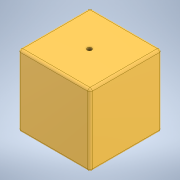
# Autodesk Inventor part: 1x2 Block v2
Saved by Autodesk Inventor 2020.1 (Build 241239000, 239)
## iProperties
Created: 2019-09-13
Part Number: 1x2 Block v2
Material: Generic
Document SubType Name: Modeling
Designer: alpha
Density: 1 g/cm^3
Appearance: Default
Author: alpha
Revision Number: ANY
Autodesk Inventor part; units mm, degrees
ref_plane "YZ Plane" through (0, 0, 0) normal (1, 0, 0) x (0, 1, 0)
ref_plane "XZ Plane" through (0, 0, 0) normal (0, 1, 0) x (-1, 0, 0)
ref_plane "XY Plane" through (0, 0, 0) normal (0, 0, 1) x (1, 0, 0)
ref_plane "Work Plane3" through (101.6, 2.54, 38.1) normal (1, 0, 0) x (0, 0, -1)
sketch "Sketch1" plane through (101.6, 2.54, 38.1) normal (1, 0, 0) x (0, 0, -1)
  line L0 (88.9, -2.54) -> (-12.7, -2.54)
  line L1 (-12.7, -2.54) -> (-12.7, 99.06)
  line L2 (-12.7, 99.06) -> (88.9, 99.06)
  line L3 (88.9, 99.06) -> (88.9, -2.54)
  point P0 (38.1, -2.54)
  constraints: 8 end point, 2 parallel, 1 horizontal, 1 perpendicular
extrude "Extrusion1" add sketch "Sketch1" along normal blind 101.6
sketch "Sketch2" plane through (101.6, 0, -50.8) normal (0, -1, 0) x (1, 0, 0)
  circle A0 centre (50.8, 50.8) radius 34.29
  point P0 (-101.6, 50.8)
  dimension "d3" = 68.58
  constraints: 1 centre point
  measures "d3" diameter of A0
extrude "Extrusion2" cut sketch "Sketch2" against normal blind 30.48
fillet "Fillet5" radius 3.175 13 edges at (152.4, 0, -50.8) (152.4, 101.6, -50.8) (101.6, 50.8, -50.8) (203.2, 50.8, -50.8) (152.4, 0, 50.8) (101.6, 0, 0) (203.2, 0, 0) (118.11, 0, 0) (152.4, 101.6, 50.8) (101.6, 101.6, 0) (203.2, 101.6, 0) (101.6, 50.8, 50.8) (203.2, 50.8, 50.8)
sketch "Sketch7" plane through (152.4, 30.48, 0) normal (0, -1, 0) x (1, 0, 0)
  point P0 (-152.4, 0)
  point P1 (0.1544, 0.9264)
hole "Hole1" at (152.5544, 30.48, 0.9264) direction (0, 1, 0) diameter 6.35 end through all
body "Solid1"
